Autodesk Fusion 360 part; units mm, degrees
(part 10 of 15)
  spline S14 degree 5 poles (-65.1777, -21.4619) (-65.1592, -21.4625) (-65.1224, -21.4637) (-65.0671, -21.4656) (-64.9935, -21.4682) (-64.9016, -21.4719) (-64.8097, -21.4758) (-64.7179, -21.48) (-64.6262, -21.4845) (-64.5346, -21.4894) (-64.443, -21.4945) (-64.3515, -21.4999) (-64.2602, -21.5056) (-64.1689, -21.5116) (-64.0777, -21.518) (-63.9866, -21.5246) (-63.8955, -21.5315) (-63.8046, -21.5388) (-63.7138, -21.5464) (-63.623, -21.5543) (-63.5324, -21.5625) (-63.4418, -21.571) (-63.3514, -21.5799) (-63.261, -21.5891) (-63.1708, -21.5986) (-63.0806, -21.6084) (-62.9906, -21.6186) (-62.9007, -21.6291) (-62.8108, -21.64) (-62.7211, -21.6512) (-62.6315, -21.6627) (-62.542, -21.6746) (-62.4527, -21.6869) (-62.3634, -21.6995) (-62.2743, -21.7125) (-62.1853, -21.7258) (-62.0964, -21.7395) (-62.0076, -21.7536) (-61.919, -21.768) (-61.8305, -21.7829) (-61.7422, -21.7981) (-61.654, -21.8137) (-61.5731, -21.8284) (-61.5099, -21.8401) (-61.4644, -21.8487) (-61.4364, -21.8541) (-61.4261, -21.8561) knots -1 -1 -1 -1 -1 -1 -0.985714 -0.971429 -0.957143 -0.942857 -0.928571 -0.914286 -0.9 -0.885714 -0.871429 -0.857143 -0.842857 -0.828571 -0.814286 -0.8 -0.785714 -0.771429 -0.757143 -0.742857 -0.728571 -0.714286 -0.7 -0.685714 -0.671429 -0.657143 -0.642857 -0.628571 -0.614286 -0.6 -0.585714 -0.571429 -0.557143 -0.542857 -0.528571 -0.514286 -0.5 -0.485714 -0.471429 -0.457143 -0.442857 -0.428571 -0.414286 -0.405839 -0.405839 -0.405839 -0.405839 -0.405839 -0.405839
  arc A14 (-60.836, -20.6774) -> (-61.4261, -21.8561) centre (2.0032, -52.8695) ccw
  spline S15 degree 5 poles (-60.836, -20.6774) (-60.8439, -20.6703) (-60.8649, -20.6511) (-60.8991, -20.6198) (-60.9463, -20.5763) (-61.0066, -20.5203) (-61.0719, -20.4591) (-61.137, -20.3975) (-61.202, -20.3355) (-61.2666, -20.2732) (-61.3311, -20.2106) (-61.3953, -20.1477) (-61.4593, -20.0844) (-61.5231, -20.0208) (-61.5867, -19.9569) (-61.6501, -19.8927) (-61.7132, -19.8282) (-61.7762, -19.7634) (-61.8389, -19.6983) (-61.9014, -19.6329) (-61.9637, -19.5672) (-62.0258, -19.5012) (-62.0877, -19.435) (-62.1494, -19.3684) (-62.2109, -19.3016) (-62.2722, -19.2345) (-62.3333, -19.1671) (-62.3942, -19.0995) (-62.4549, -19.0316) (-62.5154, -18.9634) (-62.5757, -18.8949) (-62.6359, -18.8262) (-62.6958, -18.7573) (-62.7555, -18.6881) (-62.815, -18.6186) (-62.8744, -18.5489) (-62.9335, -18.4789) (-62.9925, -18.4087) (-63.0512, -18.3382) (-63.1098, -18.2675) (-63.1682, -18.1965) (-63.2264, -18.1253) (-63.2844, -18.0539) (-63.3307, -17.9966) (-63.3653, -17.9535) (-63.3883, -17.9247) (-63.3998, -17.9103) knots 0.405839 0.405839 0.405839 0.405839 0.405839 0.405839 0.414286 0.428571 0.442857 0.457143 0.471429 0.485714 0.5 0.514286 0.528571 0.542857 0.557143 0.571429 0.585714 0.6 0.614286 0.628571 0.642857 0.657143 0.671429 0.685714 0.7 0.714286 0.728571 0.742857 0.757143 0.771429 0.785714 0.8 0.814286 0.828571 0.842857 0.857143 0.871429 0.885714 0.9 0.914286 0.928571 0.942857 0.957143 0.971429 0.985714 1 1 1 1 1 1
  arc A15 (-62.7659, -16.7493) -> (-63.3998, -17.9103) centre (2.0032, -52.8695) ccw
  spline S16 degree 5 poles (-62.7659, -16.7493) (-62.7476, -16.7512) (-62.7109, -16.755) (-62.6559, -16.7608) (-62.5827, -16.7687) (-62.4912, -16.7789) (-62.3999, -16.7894) (-62.3086, -16.8002) (-62.2174, -16.8112) (-62.1264, -16.8226) (-62.0354, -16.8342) (-61.9446, -16.8461) (-61.8539, -16.8583) (-61.7632, -16.8709) (-61.6727, -16.8837) (-61.5823, -16.8968) (-61.492, -16.9102) (-61.4018, -16.924) (-61.3118, -16.938) (-61.2218, -16.9523) (-61.132, -16.967) (-61.0423, -16.982) (-60.9527, -16.9973) (-60.8632, -17.0129) (-60.7739, -17.0288) (-60.6847, -17.0451) (-60.5956, -17.0616) (-60.5066, -17.0785) (-60.4178, -17.0958) (-60.3291, -17.1134) (-60.2406, -17.1313) (-60.1522, -17.1495) (-60.0639, -17.1681) (-59.9758, -17.1871) (-59.8878, -17.2063) (-59.8, -17.226) (-59.7123, -17.246) (-59.6248, -17.2664) (-59.5374, -17.2871) (-59.4502, -17.3082) (-59.3631, -17.3297) (-59.2763, -17.3516) (-59.1966, -17.372) (-59.1345, -17.3882) (-59.0897, -17.4) (-59.0622, -17.4074) (-59.052, -17.4101) knots -1 -1 -1 -1 -1 -1 -0.985714 -0.971429 -0.957143 -0.942857 -0.928571 -0.914286 -0.9 -0.885714 -0.871429 -0.857143 -0.842857 -0.828571 -0.814286 -0.8 -0.785714 -0.771429 -0.757143 -0.742857 -0.728571 -0.714286 -0.7 -0.685714 -0.671429 -0.657143 -0.642857 -0.628571 -0.614286 -0.6 -0.585714 -0.571429 -0.557143 -0.542857 -0.528571 -0.514286 -0.5 -0.485714 -0.471429 -0.457143 -0.442857 -0.428571 -0.414286 -0.405839 -0.405839 -0.405839 -0.405839 -0.405839 -0.405839
  arc A16 (-58.3794, -16.2765) -> (-59.052, -17.4101) centre (2.0032, -52.8695) ccw
  spline S17 degree 5 poles (-58.3794, -16.2765) (-58.3867, -16.2688) (-58.4063, -16.2482) (-58.4381, -16.2146) (-58.4822, -16.1678) (-58.5383, -16.1077) (-58.5991, -16.0419) (-58.6596, -15.9758) (-58.72, -15.9094) (-58.78, -15.8427) (-58.8399, -15.7756) (-58.8994, -15.7082) (-58.9588, -15.6406) (-59.0179, -15.5726) (-59.0767, -15.5043) (-59.1354, -15.4358) (-59.1937, -15.3669) (-59.2519, -15.2978) (-59.3098, -15.2284) (-59.3675, -15.1587) (-59.425, -15.0887) (-59.4822, -15.0185) (-59.5393, -14.9479) (-59.5961, -14.8772) (-59.6526, -14.8061) (-59.709, -14.7348) (-59.7651, -14.6633) (-59.821, -14.5914) (-59.8767, -14.5194) (-59.9322, -14.4471) (-59.9875, -14.3745) (-60.0426, -14.3017) (-60.0974, -14.2286) (-60.152, -14.1553) (-60.2065, -14.0818) (-60.2607, -14.008) (-60.3147, -13.934) (-60.3685, -13.8597) (-60.4221, -13.7852) (-60.4754, -13.7105) (-60.5286, -13.6356) (-60.5816, -13.5604) (-60.6344, -13.485) (-60.6764, -13.4246) (-60.7079, -13.3791) (-60.7288, -13.3487) (-60.7392, -13.3335) knots 0.405839 0.405839 0.405839 0.405839 0.405839 0.405839 0.414286 0.428571 0.442857 0.457143 0.471429 0.485714 0.5 0.514286 0.528571 0.542857 0.557143 0.571429 0.585714 0.6 0.614286 0.628571 0.642857 0.657143 0.671429 0.685714 0.7 0.714286 0.728571 0.742857 0.757143 0.771429 0.785714 0.8 0.814286 0.828571 0.842857 0.857143 0.871429 0.885714 0.9 0.914286 0.928571 0.942857 0.957143 0.971429 0.985714 1 1 1 1 1 1
  arc A17 (-60.0241, -12.2208) -> (-60.7392, -13.3335) centre (2.0032, -52.8695) ccw
  spline S18 degree 5 poles (-60.0241, -12.2208) (-60.0059, -12.224) (-59.9696, -12.2304) (-59.9152, -12.2401) (-59.8427, -12.2532) (-59.7522, -12.2699) (-59.6618, -12.2869) (-59.5716, -12.3041) (-59.4815, -12.3216) (-59.3914, -12.3394) (-59.3016, -12.3575) (-59.2118, -12.3759) (-59.1222, -12.3946) (-59.0327, -12.4135) (-58.9433, -12.4328) (-58.854, -12.4523) (-58.7649, -12.4721) (-58.676, -12.4923) (-58.5871, -12.5127) (-58.4984, -12.5334) (-58.4099, -12.5545) (-58.3215, -12.5758) (-58.2332, -12.5974) (-58.1451, -12.6194) (-58.0571, -12.6417) (-57.9693, -12.6642) (-57.8816, -12.6871) (-57.7941, -12.7103) (-57.7067, -12.7339) (-57.6195, -12.7577) (-57.5325, -12.7819) (-57.4456, -12.8064) (-57.3589, -12.8313) (-57.2723, -12.8564) (-57.1859, -12.882) (-57.0997, -12.9078) (-57.0137, -12.934) (-56.9278, -12.9606) (-56.8422, -12.9875) (-56.7567, -13.0148) (-56.6714, -13.0424) (-56.5863, -13.0704) (-56.5083, -13.0965) (-56.4475, -13.1171) (-56.4037, -13.1321) (-56.3768, -13.1414) (-56.3668, -13.1448) knots -1 -1 -1 -1 -1 -1 -0.985714 -0.971429 -0.957143 -0.942857 -0.928571 -0.914286 -0.9 -0.885714 -0.871429 -0.857143 -0.842857 -0.828571 -0.814286 -0.8 -0.785714 -0.771429 -0.757143 -0.742857 -0.728571 -0.714286 -0.7 -0.685714 -0.671429 -0.657143 -0.642857 -0.628571 -0.614286 -0.6 -0.585714 -0.571429 -0.557143 -0.542857 -0.528571 -0.514286 -0.5 -0.485714 -0.471429 -0.457143 -0.442857 -0.428571 -0.414286 -0.405839 -0.405839 -0.405839 -0.405839 -0.405839 -0.405839
  arc A18 (-55.615, -12.0621) -> (-56.3668, -13.1448) centre (2.0032, -52.8695) ccw
  spline S19 degree 5 poles (-55.615, -12.0621) (-55.6217, -12.0539) (-55.6398, -12.032) (-55.6692, -11.9961) (-55.7098, -11.9463) (-55.7614, -11.8824) (-55.8174, -11.8124) (-55.8731, -11.7422) (-55.9285, -11.6716) (-55.9837, -11.6008) (-56.0386, -11.5296) (-56.0932, -11.4582) (-56.1476, -11.3864) (-56.2017, -11.3144) (-56.2555, -11.2421) (-56.3091, -11.1696) (-56.3624, -11.0967) (-56.4155, -11.0236) (-56.4683, -10.9502) (-56.5209, -10.8766) (-56.5732, -10.8027) (-56.6253, -10.7286) (-56.6772, -10.6542) (-56.7288, -10.5795) (-56.7801, -10.5046) (-56.8313, -10.4295) (-56.8821, -10.3541) (-56.9328, -10.2785) (-56.9832, -10.2026) (-57.0334, -10.1265) (-57.0833, -10.0502) (-57.1331, -9.9736) (-57.1826, -9.8969) (-57.2318, -9.8198) (-57.2809, -9.7426) (-57.3297, -9.6651) (-57.3783, -9.5875) (-57.4266, -9.5096) (-57.4748, -9.4315) (-57.5227, -9.3531) (-57.5704, -9.2746) (-57.6179, -9.1958) (-57.6651, -9.1169) (-57.7027, -9.0535) (-57.7309, -9.006) (-57.7496, -8.9742) (-57.7589, -8.9583) knots 0.405839 0.405839 0.405839 0.405839 0.405839 0.405839 0.414286 0.428571 0.442857 0.457143 0.471429 0.485714 0.5 0.514286 0.528571 0.542857 0.557143 0.571429 0.585714 0.6 0.614286 0.628571 0.642857 0.657143 0.671429 0.685714 0.7 0.714286 0.728571 0.742857 0.757143 0.771429 0.785714 0.8 0.814286 0.828571 0.842857 0.857143 0.871429 0.885714 0.9 0.914286 0.928571 0.942857 0.957143 0.971429 0.985714 1 1 1 1 1 1
  arc A19 (-56.9662, -7.8993) -> (-57.7589, -8.9583) centre (2.0032, -52.8695) ccw
  spline S20 degree 5 poles (-56.9662, -7.8993) (-56.9483, -7.9038) (-56.9126, -7.9128) (-56.859, -7.9264) (-56.7876, -7.9447) (-56.6985, -7.9678) (-56.6096, -7.9911) (-56.5208, -8.0148) (-56.4321, -8.0387) (-56.3436, -8.0629) (-56.2553, -8.0873) (-56.167, -8.1121) (-56.079, -8.1371) (-55.991, -8.1624) (-55.9033, -8.1879) (-55.8157, -8.2138) (-55.7282, -8.2399) (-55.6409, -8.2664) (-55.5537, -8.2931) (-55.4667, -8.3201) (-55.3799, -8.3474) (-55.2932, -8.3749) (-55.2067, -8.4028) (-55.1204, -8.431) (-55.0342, -8.4595) (-54.9483, -8.4883) (-54.8624, -8.5174) (-54.7768, -8.5468) (-54.6913, -8.5765) (-54.606, -8.6065) (-54.5209, -8.6368) (-54.436, -8.6675) (-54.3513, -8.6984) (-54.2668, -8.7297) (-54.1824, -8.7613) (-54.0983, -8.7933) (-54.0144, -8.8256) (-53.9306, -8.8582) (-53.8471, -8.8911) (-53.7638, -8.9244) (-53.6807, -8.9581) (-53.5978, -8.9921) (-53.5219, -9.0236) (-53.4627, -9.0486) (-53.42, -9.0667) (-53.3938, -9.0778) (-53.3841, -9.082) knots -1 -1 -1 -1 -1 -1 -0.985714 -0.971429 -0.957143 -0.942857 -0.928571 -0.914286 -0.9 -0.885714 -0.871429 -0.857143 -0.842857 -0.828571 -0.814286 -0.8 -0.785714 -0.771429 -0.757143 -0.742857 -0.728571 -0.714286 -0.7 -0.685714 -0.671429 -0.657143 -0.642857 -0.628571 -0.614286 -0.6 -0.585714 -0.571429 -0.557143 -0.542857 -0.528571 -0.514286 -0.5 -0.485714 -0.471429 -0.457143 -0.442857 -0.428571 -0.414286 -0.405839 -0.405839 -0.405839 -0.405839 -0.405839 -0.405839
  arc A20 (-52.557, -8.0556) -> (-53.3841, -9.082) centre (2.0032, -52.8695) ccw
  spline S21 degree 5 poles (-52.557, -8.0556) (-52.5632, -8.047) (-52.5796, -8.0238) (-52.6064, -7.986) (-52.6433, -7.9334) (-52.6903, -7.8659) (-52.7411, -7.7922) (-52.7917, -7.7181) (-52.8419, -7.6438) (-52.8919, -7.5692) (-52.9416, -7.4943) (-52.9909, -7.4191) (-53.04, -7.3437) (-53.0889, -7.268) (-53.1374, -7.1921) (-53.1857, -7.1159) (-53.2337, -7.0394) (-53.2814, -6.9627) (-53.3289, -6.8857) (-53.3761, -6.8085) (-53.423, -6.7311) (-53.4696, -6.6534) (-53.516, -6.5755) (-53.5622, -6.4974) (-53.6081, -6.419) (-53.6537, -6.3404) (-53.6991, -6.2616) (-53.7442, -6.1826) (-53.7891, -6.1033) (-53.8337, -6.0238) (-53.8781, -5.9441) (-53.9222, -5.8642) (-53.9661, -5.7841) (-54.0098, -5.7037) (-54.0532, -5.6232) (-54.0963, -5.5425) (-54.1393, -5.4615) (-54.1819, -5.3804) (-54.2244, -5.299) (-54.2666, -5.2175) (-54.3086, -5.1357) (-54.3503, -5.0538) (-54.3918, -4.9717) (-54.4248, -4.9058) (-54.4495, -4.8563) (-54.4659, -4.8233) (-54.4741, -4.8068) knots 0.405839 0.405839 0.405839 0.405839 0.405839 0.405839 0.414286 0.428571 0.442857 0.457143 0.471429 0.485714 0.5 0.514286 0.528571 0.542857 0.557143 0.571429 0.585714 0.6 0.614286 0.628571 0.642857 0.657143 0.671429 0.685714 0.7 0.714286 0.728571 0.742857 0.757143 0.771429 0.785714 0.8 0.814286 0.828571 0.842857 0.857143 0.871429 0.885714 0.9 0.914286 0.928571 0.942857 0.957143 0.971429 0.985714 1 1 1 1 1 1
  arc A21 (-53.6078, -3.8071) -> (-54.4741, -4.8068) centre (2.0032, -52.8695) ccw
  spline S22 degree 5 poles (-53.6078, -3.8071) (-53.5903, -3.8128) (-53.5553, -3.8244) (-53.5028, -3.8417) (-53.4329, -3.865) (-53.3457, -3.8944) (-53.2587, -3.9241) (-53.1718, -3.954) (-53.0851, -3.9842) (-52.9985, -4.0146) (-52.9121, -4.0453) (-52.8259, -4.0763) (-52.7398, -4.1075) (-52.6539, -4.139) (-52.5682, -4.1708) (-52.4826, -4.2028) (-52.3973, -4.2351) (-52.3121, -4.2677) (-52.227, -4.3006) (-52.1422, -4.3337) (-52.0575, -4.3671) (-51.9731, -4.4008) (-51.8888, -4.4348) (-51.8047, -4.4691) (-51.7207, -4.5036) (-51.637, -4.5385) (-51.5535, -4.5736) (-51.4702, -4.6091) (-51.3871, -4.6448) (-51.3041, -4.6808) (-51.2214, -4.7171) (-51.1389, -4.7538) (-51.0566, -4.7907) (-50.9745, -4.8279) (-50.8927, -4.8655) (-50.811, -4.9033) (-50.7296, -4.9415) (-50.6484, -4.98) (-50.5674, -5.0189) (-50.4867, -5.058) (-50.4062, -5.0975) (-50.326, -5.1374) (-50.2525, -5.1742) (-50.1952, -5.2033) (-50.1539, -5.2244) (-50.1286, -5.2374) (-50.1192, -5.2422) knots -1 -1 -1 -1 -1 -1 -0.985714 -0.971429 -0.957143 -0.942857 -0.928571 -0.914286 -0.9 -0.885714 -0.871429 -0.857143 -0.842857 -0.828571 -0.814286 -0.8 -0.785714 -0.771429 -0.757143 -0.742857 -0.728571 -0.714286 -0.7 -0.685714 -0.671429 -0.657143 -0.642857 -0.628571 -0.614286 -0.6 -0.585714 -0.571429 -0.557143 -0.542857 -0.528571 -0.514286 -0.5 -0.485714 -0.471429 -0.457143 -0.442857 -0.428571 -0.414286 -0.405839 -0.405839 -0.405839 -0.405839 -0.405839 -0.405839
  arc A22 (-49.221, -4.2775) -> (-50.1192, -5.2422) centre (2.0032, -52.8695) ccw
  spline S23 degree 5 poles (-49.221, -4.2775) (-49.2265, -4.2685) (-49.2413, -4.2442) (-49.2653, -4.2045) (-49.2984, -4.1495) (-49.3404, -4.0788) (-49.3859, -4.0016) (-49.431, -3.9241) (-49.4758, -3.8464) (-49.5203, -3.7684) (-49.5645, -3.6902) (-49.6084, -3.6117) (-49.652, -3.533) (-49.6953, -3.454) (-49.7383, -3.3748) (-49.781, -3.2953) (-49.8235, -3.2156) (-49.8656, -3.1357) (-49.9074, -3.0556) (-49.949, -2.9752) (-49.9903, -2.8946) (-50.0313, -2.8138) (-50.072, -2.7328) (-50.1125, -2.6515) (-50.1527, -2.5701) (-50.1926, -2.4885) (-50.2322, -2.4066) (-50.2716, -2.3245) (-50.3107, -2.2423) (-50.3495, -2.1598) (-50.3881, -2.0771) (-50.4264, -1.9943) (-50.4645, -1.9112) (-50.5023, -1.828) (-50.5398, -1.7446) (-50.5771, -1.661) (-50.6142, -1.5772) (-50.651, -1.4932) (-50.6875, -1.409) (-50.7238, -1.3246) (-50.7598, -1.2401) (-50.7956, -1.1554) (-50.8311, -1.0705) (-50.8594, -1.0025) (-50.8804, -0.9514) (-50.8944, -0.9173) (-50.9014, -0.9002) knots 0.405839 0.405839 0.405839 0.405839 0.405839 0.405839 0.414286 0.428571 0.442857 0.457143 0.471429 0.485714 0.5 0.514286 0.528571 0.542857 0.557143 0.571429 0.585714 0.6 0.614286 0.628571 0.642857 0.657143 0.671429 0.685714 0.7 0.714286 0.728571 0.742857 0.757143 0.771429 0.785714 0.8 0.814286 0.828571 0.842857 0.857143 0.871429 0.885714 0.9 0.914286 0.928571 0.942857 0.957143 0.971429 0.985714 1 1 1 1 1 1
  arc A23 (-49.9661, 0.0351) -> (-50.9014, -0.9002) centre (2.0032, -52.8695) ccw
  spline S24 degree 5 poles (-49.9661, 0.0351) (-49.949, 0.0282) (-49.9149, 0.0142) (-49.8638, -0.0069) (-49.7957, -0.0351) (-49.7109, -0.0707) (-49.6261, -0.1065) (-49.5416, -0.1425) (-49.4573, -0.1788) (-49.3731, -0.2153) (-49.2891, -0.2521) (-49.2053, -0.2891) (-49.1217, -0.3264) (-49.0383, -0.364) (-48.955, -0.4018) (-48.872, -0.4398) (-48.7891, -0.4782) (-48.7065, -0.5167) (-48.624, -0.5556) (-48.5417, -0.5947) (-48.4597, -0.6341) (-48.3778, -0.6737) (-48.2962, -0.7136) (-48.2147, -0.7538) (-48.1335, -0.7942) (-48.0525, -0.835) (-47.9717, -0.876) (-47.8911, -0.9173) (-47.8107, -0.9588) (-47.7306, -1.0007) (-47.6506, -1.0428) (-47.571, -1.0852) (-47.4915, -1.1279) (-47.4123, -1.1709) (-47.3333, -1.2142) (-47.2546, -1.2578) (-47.1761, -1.3017) (-47.0978, -1.3459) (-47.0199, -1.3904) (-46.9421, -1.4353) (-46.8647, -1.4804) (-46.7875, -1.5259) (-46.7168, -1.5679) (-46.6617, -1.601) (-46.6221, -1.625) (-46.5978, -1.6397) (-46.5887, -1.6452) knots -1 -1 -1 -1 -1 -1 -0.985714 -0.971429 -0.957143 -0.942857 -0.928571 -0.914286 -0.9 -0.885714 -0.871429 -0.857143 -0.842857 -0.828571 -0.814286 -0.8 -0.785714 -0.771429 -0.757143 -0.742857 -0.728571 -0.714286 -0.7 -0.685714 -0.671429 -0.657143 -0.642857 -0.628571 -0.614286 -0.6 -0.585714 -0.571429 -0.557143 -0.542857 -0.528571 -0.514286 -0.5 -0.485714 -0.471429 -0.457143 -0.442857 -0.428571 -0.414286 -0.405839 -0.405839 -0.405839 -0.405839 -0.405839 -0.405839
  arc A24 (-45.624, -0.747) -> (-46.5887, -1.6452) centre (2.0032, -52.8695) ccw
  spline S25 degree 5 poles (-45.624, -0.747) (-45.6289, -0.7376) (-45.6419, -0.7123) (-45.663, -0.6711) (-45.692, -0.6138) (-45.7289, -0.5403) (-45.7687, -0.4601) (-45.8082, -0.3796) (-45.8474, -0.2988) (-45.8862, -0.2179) (-45.9247, -0.1367) (-45.9629, -0.0553) (-46.0008, 0.0264) (-46.0383, 0.1083) (-46.0756, 0.1903) (-46.1125, 0.2726) (-46.1491, 0.3551) (-46.1855, 0.4379) (-46.2215, 0.5208) (-46.2572, 0.6039) (-46.2926, 0.6872) (-46.3278, 0.7708) (-46.3626, 0.8545) (-46.3972, 0.9384) (-46.4314, 1.0225) (-46.4654, 1.1068) (-46.4991, 1.1913) (-46.5326, 1.2759) (-46.5657, 1.3608) (-46.5986, 1.4458) (-46.6311, 1.531) (-46.6635, 1.6164) (-46.6955, 1.7019) (-46.7273, 1.7877) (-46.7588, 1.8735) (-46.79, 1.9596) (-46.821, 2.0458) (-46.8517, 2.1322) (-46.8821, 2.2188) (-46.9123, 2.3055) (-46.9422, 2.3924) (-46.9718, 2.4794) (-47.0012, 2.5666) (-47.0245, 2.6365) (-47.0419, 2.689) (-47.0534, 2.724) (-47.0592, 2.7416) knots 0.405839 0.405839 0.405839 0.405839 0.405839 0.405839 0.414286 0.428571 0.442857 0.457143 0.471429 0.485714 0.5 0.514286 0.528571 0.542857 0.557143 0.571429 0.585714 0.6 0.614286 0.628571 0.642857 0.657143 0.671429 0.685714 0.7 0.714286 0.728571 0.742857 0.757143 0.771429 0.785714 0.8 0.814286 0.828571 0.842857 0.857143 0.871429 0.885714 0.9 0.914286 0.928571 0.942857 0.957143 0.971429 0.985714 1 1 1 1 1 1
  arc A25 (-46.0595, 3.6078) -> (-47.0592, 2.7416) centre (2.0032, -52.8695) ccw
  spline S26 degree 5 poles (-46.0595, 3.6078) (-46.043, 3.5996) (-46.0099, 3.5832) (-45.9605, 3.5586) (-45.8946, 3.5255) (-45.8125, 3.484) (-45.7305, 3.4423) (-45.6488, 3.4003) (-45.5672, 3.3581) (-45.4859, 3.3157) (-45.4047, 3.273) (-45.3238, 3.2301) (-45.2431, 3.1869) (-45.1625, 3.1435) (-45.0822, 3.0999) (-45.0021, 3.056) (-44.9222, 3.0118) (-44.8425, 2.9675) (-44.763, 2.9228) (-44.6837, 2.878) (-44.6047, 2.8328) (-44.5258, 2.7874) (-44.4472, 2.7418) (-44.3689, 2.6959) (-44.2907, 2.6498) (-44.2128, 2.6034) (-44.1352, 2.5567) (-44.0577, 2.5098) (-43.9805, 2.4626) (-43.9036, 2.4151) (-43.8269, 2.3674) (-43.7504, 2.3194) (-43.6742, 2.2711) (-43.5983, 2.2226) (-43.5226, 2.1738) (-43.4471, 2.1247) (-43.372, 2.0753) (-43.2971, 2.0256) (-43.2225, 1.9757) (-43.1481, 1.9254) (-43.0741, 1.8749) (-43.0003, 1.824) (-42.9329, 1.7771) (-42.8803, 1.7401) (-42.8425, 1.7134) (-42.8193, 1.6969) (-42.8106, 1.6908) knots -1 -1 -1 -1 -1 -1 -0.985714 -0.971429 -0.957143 -0.942857 -0.928571 -0.914286 -0.9 -0.885714 -0.871429 -0.857143 -0.842857 -0.828571 -0.814286 -0.8 -0.785714 -0.771429 -0.757143 -0.742857 -0.728571 -0.714286 -0.7 -0.685714 -0.671429 -0.657143 -0.642857 -0.628571 -0.614286 -0.6 -0.585714 -0.571429 -0.557143 -0.542857 -0.528571 -0.514286 -0.5 -0.485714 -0.471429 -0.457143 -0.442857 -0.428571 -0.414286 -0.405839 -0.405839 -0.405839 -0.405839 -0.405839 -0.405839
  arc A26 (-41.7843, 2.5179) -> (-42.8106, 1.6908) centre (2.0032, -52.8695) ccw
  spline S27 degree 5 poles (-41.7843, 2.5179) (-41.7885, 2.5276) (-41.7996, 2.5537) (-41.8177, 2.5964) (-41.8426, 2.6556) (-41.8742, 2.7315) (-41.9082, 2.8144) (-41.9418, 2.8975) (-41.9751, 2.9808) (-42.0081, 3.0644) (-42.0407, 3.1481) (-42.073, 3.232) (-42.1049, 3.3162) (-42.1365, 3.4005) (-42.1678, 3.485) (-42.1988, 3.5698) (-42.2295, 3.6547) (-42.2598, 3.7398) (-42.2898, 3.8251) (-42.3195, 3.9105) (-42.3489, 3.9962) (-42.378, 4.082) (-42.4068, 4.168) (-42.4353, 4.2541) (-42.4634, 4.3405) (-42.4913, 4.427) (-42.5189, 4.5136) (-42.5462, 4.6005) (-42.5732, 4.6875) (-42.5999, 4.7746) (-42.6263, 4.8619) (-42.6525, 4.9494) (-42.6783, 5.037) (-42.7039, 5.1248) (-42.7292, 5.2127) (-42.7542, 5.3008) (-42.7789, 5.389) (-42.8034, 5.4774) (-42.8276, 5.5659) (-42.8515, 5.6545) (-42.8751, 5.7433) (-42.8985, 5.8323) (-42.9216, 5.9213) (-42.9399, 5.9927) (-42.9534, 6.0463) (-42.9624, 6.0821) (-42.9669, 6.0999) knots 0.405839 0.405839 0.405839 0.405839 0.405839 0.405839 0.414286 0.428571 0.442857 0.457143 0.471429 0.485714 0.5 0.514286 0.528571 0.542857 0.557143 0.571429 0.585714 0.6 0.614286 0.628571 0.642857 0.657143 0.671429 0.685714 0.7 0.714286 0.728571 0.742857 0.757143 0.771429 0.785714 0.8 0.814286 0.828571 0.842857 0.857143 0.871429 0.885714 0.9 0.914286 0.928571 0.942857 0.957143 0.971429 0.985714 1 1 1 1 1 1
  arc A27 (-41.908, 6.8927) -> (-42.9669, 6.0999) centre (2.0032, -52.8695) ccw
  spline S28 degree 5 poles (-41.908, 6.8927) (-41.8921, 6.8833) (-41.8603, 6.8646) (-41.8127, 6.8365) (-41.7494, 6.7988) (-41.6704, 6.7516) (-41.5917, 6.7041) (-41.5131, 6.6564) (-41.4348, 6.6085) (-41.3567, 6.5604) (-41.2788, 6.512) (-41.2011, 6.4634) (-41.1237, 6.4146) (-41.0464, 6.3656) (-40.9694, 6.3163) (-40.8926, 6.2668) (-40.8161, 6.2171) (-40.7397, 6.1671) (-40.6636, 6.1169) (-40.5878, 6.0665) (-40.5122, 6.0159) (-40.4368, 5.965) (-40.3616, 5.9139) (-40.2867, 5.8625) (-40.2121, 5.8109) (-40.1377, 5.7591) (-40.0635, 5.707) (-39.9896, 5.6546) (-39.916, 5.6021) (-39.8426, 5.5492) (-39.7695, 5.4962) (-39.6967, 5.4428) (-39.6241, 5.3892) (-39.5518, 5.3354) (-39.4798, 5.2813) (-39.4081, 5.2269) (-39.3367, 5.1723) (-39.2655, 5.1174) (-39.1946, 5.0623) (-39.1241, 5.0069) (-39.0538, 4.9512) (-38.9839, 4.8952) (-38.9199, 4.8435) (-38.8701, 4.8029) (-38.8343, 4.7736) (-38.8123, 4.7555) (-38.8042, 4.7487) knots -1 -1 -1 -1 -1 -1 -0.985714 -0.971429 -0.957143 -0.942857 -0.928571 -0.914286 -0.9 -0.885714 -0.871429 -0.857143 -0.842857 -0.828571 -0.814286 -0.8 -0.785714 -0.771429 -0.757143 -0.742857 -0.728571 -0.714286 -0.7 -0.685714 -0.671429 -0.657143 -0.642857 -0.628571 -0.614286 -0.6 -0.585714 -0.571429 -0.557143 -0.542857 -0.528571 -0.514286 -0.5 -0.485714 -0.471429 -0.457143 -0.442857 -0.428571 -0.414286 -0.405839 -0.405839 -0.405839 -0.405839 -0.405839 -0.405839
  arc A28 (-37.7214, 5.5005) -> (-38.8042, 4.7487) centre (2.0032, -52.8695) ccw
  spline S29 degree 5 poles (-37.7214, 5.5005) (-37.7249, 5.5105) (-37.7342, 5.5374) (-37.7492, 5.5812) (-37.7698, 5.6421) (-37.7958, 5.72) (-37.8238, 5.8051) (-37.8515, 5.8904) (-37.8788, 5.9759) (-37.9057, 6.0616) (-37.9322, 6.1474) (-37.9584, 6.2335) (-37.9843, 6.3197) (-38.0098, 6.406) (-38.035, 6.4926) (-38.0599, 6.5793) (-38.0844, 6.6662) (-38.1086, 6.7532) (-38.1324, 6.8404) (-38.1559, 6.9278) (-38.1791, 7.0153) (-38.202, 7.103) (-38.2246, 7.1908) (-38.2469, 7.2788) (-38.2688, 7.3669) (-38.2905, 7.4552) (-38.3118, 7.5436) (-38.3328, 7.6322) (-38.3536, 7.7209) (-38.374, 7.8097) (-38.3941, 7.8987) (-38.414, 7.9878) (-38.4335, 8.077) (-38.4527, 8.1664) (-38.4717, 8.2559) (-38.4904, 8.3455) (-38.5087, 8.4353) (-38.5268, 8.5252) (-38.5446, 8.6152) (-38.5622, 8.7053) (-38.5794, 8.7956) (-38.5964, 8.886) (-38.613, 8.9764) (-38.6262, 9.0489) (-38.6359, 9.1034) (-38.6423, 9.1397) (-38.6455, 9.1578) knots 0.405839 0.405839 0.405839 0.405839 0.405839 0.405839 0.414286 0.428571 0.442857 0.457143 0.471429 0.485714 0.5 0.514286 0.528571 0.542857 0.557143 0.571429 0.585714 0.6 0.614286 0.628571 0.642857 0.657143 0.671429 0.685714 0.7 0.714286 0.728571 0.742857 0.757143 0.771429 0.785714 0.8 0.814286 0.828571 0.842857 0.857143 0.871429 0.885714 0.9 0.914286 0.928571 0.942857 0.957143 0.971429 0.985714 1 1 1 1 1 1
  arc A29 (-37.5327, 9.873) -> (-38.6455, 9.1578) centre (2.0032, -52.8695) ccw
  spline S30 degree 5 poles (-37.5327, 9.873) (-37.5175, 9.8625) (-37.4872, 9.8416) (-37.4417, 9.8101) (-37.3812, 9.7681) (-37.3058, 9.7153) (-37.2307, 9.6624) (-37.1557, 9.6092) (-37.081, 9.5558) (-37.0065, 9.5022) (-36.9323, 9.4484) (-36.8583, 9.3944) (-36.7845, 9.3402) (-36.711, 9.2858) (-36.6377, 9.2311) (-36.5646, 9.1763) (-36.4918, 9.1212) (-36.4192, 9.066) (-36.3469, 9.0105) (-36.2748, 8.9548) (-36.203, 8.8989) (-36.1314, 8.8427) (-36.0601, 8.7864) (-35.9891, 8.7298) (-35.9183, 8.673) (-35.8478, 8.616) (-35.7776, 8.5587) (-35.7076, 8.5013) (-35.6379, 8.4436) (-35.5685, 8.3856) (-35.4994, 8.3275) (-35.4305, 8.2691) (-35.3619, 8.2105) (-35.2937, 8.1516) (-35.2257, 8.0925) (-35.158, 8.0332) (-35.0907, 7.9736) (-35.0236, 7.9138) (-34.9569, 7.8537) (-34.8904, 7.7934) (-34.8243, 7.7328) (-34.7586, 7.672) (-34.6985, 7.6159) (-34.6517, 7.5719) (-34.618, 7.54) (-34.5974, 7.5204) (-34.5898, 7.5131) knots -1 -1 -1 -1 -1 -1 -0.985714 -0.971429 -0.957143 -0.942857 -0.928571 -0.914286 -0.9 -0.885714 -0.871429 -0.857143 -0.842857 -0.828571 -0.814286 -0.8 -0.785714 -0.771429 -0.757143 -0.742857 -0.728571 -0.714286 -0.7 -0.685714 -0.671429 -0.657143 -0.642857 -0.628571 -0.614286 -0.6 -0.585714 -0.571429 -0.557143 -0.542857 -0.528571 -0.514286 -0.5 -0.485714 -0.471429 -0.457143 -0.442857 -0.428571 -0.414286 -0.405839 -0.405839 -0.405839 -0.405839 -0.405839 -0.405839
  arc A30 (-33.4562, 8.1857) -> (-34.5898, 7.5131) centre (2.0032, -52.8695) ccw
  spline S31 degree 5 poles (-33.4562, 8.1857) (-33.4589, 8.1959) (-33.4662, 8.2234) (-33.4781, 8.2682) (-33.4943, 8.3304) (-33.5147, 8.41) (-33.5366, 8.4969) (-33.5581, 8.5839) (-33.5792, 8.6711) (-33.5999, 8.7585) (-33.6203, 8.846) (-33.6403, 8.9337) (-33.6599, 9.0215) (-33.6792, 9.1095) (-33.6982, 9.1976) (-33.7168, 9.2859) (-33.735, 9.3743) (-33.7529, 9.4629) (-33.7705, 9.5515) (-33.7877, 9.6404) (-33.8046, 9.7293) (-33.8212, 9.8184) (-33.8375, 9.9076) (-33.8534, 9.997) (-33.869, 10.0864) (-33.8843, 10.176) (-33.8993, 10.2657) (-33.9139, 10.3556) (-33.9283, 10.4455) (-33.9423, 10.5356) (-33.956, 10.6258) (-33.9695, 10.716) (-33.9826, 10.8065) (-33.9954, 10.897) (-34.0079, 10.9876) (-34.0202, 11.0783) (-34.0321, 11.1692) (-34.0437, 11.2601) (-34.0551, 11.3512) (-34.0661, 11.4423) (-34.0769, 11.5336) (-34.0873, 11.6249) (-34.0975, 11.7164) (-34.1054, 11.7896) (-34.1113, 11.8446) (-34.1151, 11.8813) (-34.117, 11.8996) knots 0.405839 0.405839 0.405839 0.405839 0.405839 0.405839 0.414286 0.428571 0.442857 0.457143 0.471429 0.485714 0.5 0.514286 0.528571 0.542857 0.557143 0.571429 0.585714 0.6 0.614286 0.628571 0.642857 0.657143 0.671429 0.685714 0.7 0.714286 0.728571 0.742857 0.757143 0.771429 0.785714 0.8 0.814286 0.828571 0.842857 0.857143 0.871429 0.885714 0.9 0.914286 0.928571 0.942857 0.957143 0.971429 0.985714 1 1 1 1 1 1
  arc A31 (-32.956, 12.5336) -> (-34.117, 11.8996) centre (2.0032, -52.8695) ccw
  spline S32 degree 5 poles (-32.956, 12.5336) (-32.9416, 12.5221) (-32.9128, 12.499) (-32.8697, 12.4644) (-32.8124, 12.4182) (-32.7409, 12.3601) (-32.6697, 12.3019) (-32.5988, 12.2436) (-32.5281, 12.185) (-32.4576, 12.1262) (-32.3874, 12.0673) (-32.3174, 12.0081) (-32.2477, 11.9488) (-32.1782, 11.8892) (-32.109, 11.8295) (-32.04, 11.7696) (-31.9713, 11.7095) (-31.9029, 11.6492) (-31.8347, 11.5887) (-31.7668, 11.528) (-31.6992, 11.4671) (-31.6318, 11.406) (-31.5647, 11.3447) (-31.4979, 11.2832) (-31.4313, 11.2215) (-31.365, 11.1596) (-31.2991, 11.0975) (-31.2334, 11.0352) (-31.168, 10.9726) (-31.1029, 10.9099) (-31.0381, 10.847) (-30.9736, 10.7838) (-30.9093, 10.7204) (-30.8455, 10.6569) (-30.7819, 10.5931) (-30.7186, 10.5291) (-30.6557, 10.4648) (-30.593, 10.4004) (-30.5308, 10.3357) (-30.4688, 10.2708) (-30.4072, 10.2057) (-30.3459, 10.1403) (-30.29, 10.0801) (-30.2465, 10.0328) (-30.2152, 9.9986) (-30.196, 9.9776) (-30.1889, 9.9698) knots -1 -1 -1 -1 -1 -1 -0.985714 -0.971429 -0.957143 -0.942857 -0.928571 -0.914286 -0.9 -0.885714 -0.871429 -0.857143 -0.842857 -0.828571 -0.814286 -0.8 -0.785714 -0.771429 -0.757143 -0.742857 -0.728571 -0.714286 -0.7 -0.685714 -0.671429 -0.657143 -0.642857 -0.628571 -0.614286 -0.6 -0.585714 -0.571429 -0.557143 -0.542857 -0.528571 -0.514286 -0.5 -0.485714 -0.471429 -0.457143 -0.442857 -0.428571 -0.414286 -0.405839 -0.405839 -0.405839 -0.405839 -0.405839 -0.405839
  arc A32 (-29.0102, 10.5598) -> (-30.1889, 9.9698) centre (2.0032, -52.8695) ccw
  spline S33 degree 5 poles (-29.0102, 10.5598) (-29.0122, 10.5702) (-29.0175, 10.5981) (-29.0261, 10.6436) (-29.0379, 10.7068) (-29.0526, 10.7877) (-29.0682, 10.8759) (-29.0834, 10.9643) (-29.0982, 11.0528) (-29.1127, 11.1414) (-29.1268, 11.2301) (-29.1405, 11.319) (-29.1538, 11.408) (-29.1668, 11.4972) (-29.1794, 11.5864) (-29.1916, 11.6758) (-29.2035, 11.7653) (-29.2151, 11.8549) (-29.2263, 11.9446) (-29.2371, 12.0344) (-29.2477, 12.1243) (-29.2578, 12.2144) (-29.2677, 12.3045) (-29.2772, 12.3948) (-29.2864, 12.4851) (-29.2952, 12.5756) (-29.3038, 12.6661) (-29.312, 12.7568) (-29.3199, 12.8475) (-29.3275, 12.9383) (-29.3347, 13.0293) (-29.3417, 13.1203) (-29.3483, 13.2114) (-29.3546, 13.3026) (-29.3607, 13.3939) (-29.3664, 13.4853) (-29.3718, 13.5767) (-29.3769, 13.6683) (-29.3817, 13.7599) (-29.3862, 13.8516) (-29.3905, 13.9434) (-29.3944, 14.0353) (-29.398, 14.1272) (-29.4007, 14.2009) (-29.4026, 14.2561) (-29.4038, 14.293) (-29.4044, 14.3114) knots 0.405839 0.405839 0.405839 0.405839 0.405839 0.405839 0.414286 0.428571 0.442857 0.457143 0.471429 0.485714 0.5 0.514286 0.528571 0.542857 0.557143 0.571429 0.585714 0.6 0.614286 0.628571 0.642857 0.657143 0.671429 0.685714 0.7 0.714286 0.728571 0.742857 0.757143 0.771429 0.785714 0.8 0.814286 0.828571 0.842857 0.857143 0.871429 0.885714 0.9 0.914286 0.928571 0.942857 0.957143 0.971429 0.985714 1 1 1 1 1 1
  arc A33 (-28.2011, 14.8609) -> (-29.4044, 14.3114) centre (2.0032, -52.8695) ccw
  spline S34 degree 5 poles (-28.2011, 14.8609) (-28.1876, 14.8484) (-28.1605, 14.8234) (-28.12, 14.7858) (-28.0661, 14.7355) (-27.999, 14.6726) (-27.9321, 14.6094) (-27.8655, 14.5461) (-27.7992, 14.4827) (-27.7331, 14.419) (-27.6672, 14.3552) (-27.6017, 14.2912) (-27.5363, 14.227) (-27.4713, 14.1627) (-27.4065, 14.0982) (-27.342, 14.0335) (-27.2778, 13.9687) (-27.2138, 13.9036) (-27.1501, 13.8384) (-27.0867, 13.773) (-27.0236, 13.7075) (-26.9607, 13.6417) (-26.8982, 13.5758) (-26.8359, 13.5097) (-26.7739, 13.4434) (-26.7122, 13.3769) (-26.6509, 13.3102) (-26.5898, 13.2434) (-26.529, 13.1764) (-26.4685, 13.1092) (-26.4084, 13.0418) (-26.3486, 12.9742) (-26.289, 12.9064) (-26.2298, 12.8384) (-26.171, 12.7702) (-26.1124, 12.7019) (-26.0542, 12.6333) (-25.9964, 12.5646) (-25.9389, 12.4956) (-25.8817, 12.4264) (-25.8249, 12.3571) (-25.7684, 12.2875) (-25.7169, 12.2234) (-25.6769, 12.1732) (-25.6481, 12.1369) (-25.6305, 12.1145) (-25.624, 12.1062) knots -1 -1 -1 -1 -1 -1 -0.985714 -0.971429 -0.957143 -0.942857 -0.928571 -0.914286 -0.9 -0.885714 -0.871429 -0.857143 -0.842857 -0.828571 -0.814286 -0.8 -0.785714 -0.771429 -0.757143 -0.742857 -0.728571 -0.714286 -0.7 -0.685714 -0.671429 -0.657143 -0.642857 -0.628571 -0.614286 -0.6 -0.585714 -0.571429 -0.557143 -0.542857 -0.528571 -0.514286 -0.5 -0.485714 -0.471429 -0.457143 -0.442857 -0.428571 -0.414286 -0.405839 -0.405839 -0.405839 -0.405839 -0.405839 -0.405839
  arc A34 (-24.4062, 12.6106) -> (-25.624, 12.1062) centre (2.0032, -52.8695) ccw
  spline S35 degree 5 poles (-24.4062, 12.6106) (-24.4074, 12.6211) (-24.4108, 12.6494) (-24.4161, 12.6954) (-24.4233, 12.7593) (-24.4322, 12.841) (-24.4415, 12.9301) (-24.4504, 13.0193) (-24.4588, 13.1086) (-24.4669, 13.1981) (-24.4746, 13.2876) (-24.482, 13.3772) (-24.4889, 13.467) (-24.4955, 13.5568) (-24.5017, 13.6467) (-24.5075, 13.7367) (-24.513, 13.8268) (-24.5182, 13.917) (-24.5229, 14.0073) (-24.5273, 14.0977) (-24.5314, 14.1881) (-24.5352, 14.2787) (-24.5385, 14.3693) (-24.5416, 14.46) (-24.5443, 14.5508) (-24.5467, 14.6416) (-24.5488, 14.7326) (-24.5505, 14.8236) (-24.5519, 14.9146) (-24.553, 15.0058) (-24.5537, 15.097) (-24.5542, 15.1883) (-24.5543, 15.2796) (-24.5541, 15.3711) (-24.5536, 15.4625) (-24.5528, 15.5541) (-24.5516, 15.6457) (-24.5502, 15.7374) (-24.5485, 15.8291) (-24.5464, 15.9209) (-24.5441, 16.0128) (-24.5415, 16.1047) (-24.5385, 16.1967) (-24.536, 16.2703) (-24.5339, 16.3256) (-24.5324, 16.3624) (-24.5317, 16.3808) knots 0.405839 0.405839 0.405839 0.405839 0.405839 0.405839 0.414286 0.428571 0.442857 0.457143 0.471429 0.485714 0.5 0.514286 0.528571 0.542857 0.557143 0.571429 0.585714 0.6 0.614286 0.628571 0.642857 0.657143 0.671429 0.685714 0.7 0.714286 0.728571 0.742857 0.757143 0.771429 0.785714 0.8 0.814286 0.828571 0.842857 0.857143 0.871429 0.885714 0.9 0.914286 0.928571 0.942857 0.957143 0.971429 0.985714 1 1 1 1 1 1
  arc A35 (-23.2923, 16.8431) -> (-24.5317, 16.3808) centre (2.0032, -52.8695) ccw
  spline S36 degree 5 poles (-23.2923, 16.8431) (-23.2797, 16.8296) (-23.2545, 16.8027) (-23.2168, 16.7623) (-23.1666, 16.7084) (-23.1041, 16.6408) (-23.042, 16.5731) (-22.98, 16.5052) (-22.9184, 16.4371) (-22.857, 16.3689) (-22.7959, 16.3006) (-22.735, 16.2321) (-22.6745, 16.1634) (-22.6142, 16.0946) (-22.5542, 16.0256) (-22.4944, 15.9565) (-22.435, 15.8872) (-22.3758, 15.8178) (-22.3169, 15.7482) (-22.2584, 15.6785) (-22.2001, 15.6086) (-22.1421, 15.5385) (-22.0844, 15.4683) (-22.027, 15.3979) (-21.9699, 15.3274) (-21.9131, 15.2566) (-21.8566, 15.1858) (-21.8005, 15.1148) (-21.7447, 15.0436) (-21.6891, 14.9722) (-21.634, 14.9007) (-21.5791, 14.829) (-21.5246, 14.7571) (-21.4704, 14.6851) (-21.4165, 14.6129) (-21.363, 14.5405) (-21.3098, 14.468) (-21.257, 14.3953) (-21.2046, 14.3224) (-21.1525, 14.2494) (-21.1008, 14.1761) (-21.0494, 14.1027) (-21.0026, 14.0351) (-20.9663, 13.9821) (-20.9402, 13.9439) (-20.9242, 13.9203) (-20.9183, 13.9116) knots -1 -1 -1 -1 -1 -1 -0.985714 -0.971429 -0.957143 -0.942857 -0.928571 -0.914286 -0.9 -0.885714 -0.871429 -0.857143 -0.842857 -0.828571 -0.814286 -0.8 -0.785714 -0.771429 -0.757143 -0.742857 -0.728571 -0.714286 -0.7 -0.685714 -0.671429 -0.657143 -0.642857 -0.628571 -0.614286 -0.6 -0.585714 -0.571429 -0.557143 -0.542857 -0.528571 -0.514286 -0.5 -0.485714 -0.471429 -0.457143 -0.442857 -0.428571 -0.414286 -0.405839 -0.405839 -0.405839 -0.405839 -0.405839 -0.405839
  arc A36 (-19.6676, 14.3278) -> (-20.9183, 13.9116) centre (2.0032, -52.8695) ccw
  spline S37 degree 5 poles (-19.6676, 14.3278) (-19.6681, 14.3384) (-19.6694, 14.3668) (-19.6715, 14.4131) (-19.6741, 14.4773) (-19.6771, 14.5594) (-19.68, 14.649) (-19.6825, 14.7386) (-19.6846, 14.8283) (-19.6863, 14.9181) (-19.6876, 15.0079) (-19.6885, 15.0979) (-19.689, 15.1879) (-19.6892, 15.2779) (-19.689, 15.3681) (-19.6884, 15.4583) (-19.6874, 15.5486) (-19.6861, 15.6389) (-19.6844, 15.7293) (-19.6824, 15.8197) (-19.68, 15.9102) (-19.6772, 16.0008) (-19.6742, 16.0914) (-19.6707, 16.1821) (-19.667, 16.2729) (-19.6629, 16.3637) (-19.6584, 16.4545) (-19.6537, 16.5454) (-19.6486, 16.6363) (-19.6431, 16.7273) (-19.6374, 16.8184) (-19.6313, 16.9095) (-19.6249, 17.0006) (-19.6182, 17.0918) (-19.6112, 17.183) (-19.6038, 17.2742) (-19.5962, 17.3655) (-19.5882, 17.4569) (-19.5799, 17.5483) (-19.5713, 17.6397) (-19.5625, 17.7312) (-19.5533, 17.8226) (-19.5438, 17.9142) (-19.536, 17.9874) (-19.53, 18.0424) (-19.5259, 18.079) (-19.5238, 18.0974) knots 0.405839 0.405839 0.405839 0.405839 0.405839 0.405839 0.414286 0.428571 0.442857 0.457143 0.471429 0.485714 0.5 0.514286 0.528571 0.542857 0.557143 0.571429 0.585714 0.6 0.614286 0.628571 0.642857 0.657143 0.671429 0.685714 0.7 0.714286 0.728571 0.742857 0.757143 0.771429 0.785714 0.8 0.814286 0.828571 0.842857 0.857143 0.871429 0.885714 0.9 0.914286 0.928571 0.942857 0.957143 0.971429 0.985714 1 1 1 1 1 1
  arc A37 (-18.2546, 18.47) -> (-19.5238, 18.0974) centre (2.0032, -52.8695) ccw
  spline S38 degree 5 poles (-18.2546, 18.47) (-18.243, 18.4557) (-18.2198, 18.4271) (-18.185, 18.3841) (-18.1388, 18.3267) (-18.0814, 18.2548) (-18.0242, 18.1828) (-17.9672, 18.1107) (-17.9106, 18.0384) (-17.8542, 17.966) (-17.7982, 17.8935) (-17.7424, 17.8208) (-17.6868, 17.748) (-17.6316, 17.6751) (-17.5767, 17.602) (-17.522, 17.5288) (-17.4677, 17.4555) (-17.4136, 17.382) (-17.3598, 17.3084) (-17.3064, 17.2346) (-17.2532, 17.1607) (-17.2004, 17.0867) (-17.1478, 17.0126) (-17.0956, 16.9383) (-17.0437, 16.8638) (-16.9921, 16.7892) (-16.9409, 16.7145) (-16.8899, 16.6397) (-16.8393, 16.5647) (-16.789, 16.4895) (-16.7391, 16.4143) (-16.6895, 16.3388) (-16.6402, 16.2633) (-16.5913, 16.1876) (-16.5427, 16.1117) (-16.4945, 16.0357) (-16.4466, 15.9596) (-16.3991, 15.8833) (-16.352, 15.8068) (-16.3053, 15.7303) (-16.2589, 15.6535) (-16.213, 15.5766) (-16.1711, 15.5059) (-16.1386, 15.4504) (-16.1153, 15.4104) (-16.101, 15.3858) (-16.0958, 15.3766) knots -1 -1 -1 -1 -1 -1 -0.985714 -0.971429 -0.957143 -0.942857 -0.928571 -0.914286 -0.9 -0.885714 -0.871429 -0.857143 -0.842857 -0.828571 -0.814286 -0.8 -0.785714 -0.771429 -0.757143 -0.742857 -0.728571 -0.714286 -0.7 -0.685714 -0.671429 -0.657143 -0.642857 -0.628571 -0.614286 -0.6 -0.585714 -0.571429 -0.557143 -0.542857 -0.528571 -0.514286 -0.5 -0.485714 -0.471429 -0.457143 -0.442857 -0.428571 -0.414286 -0.405839 -0.405839 -0.405839 -0.405839 -0.405839 -0.405839
  arc A38 (-14.8186, 15.7026) -> (-16.0958, 15.3766) centre (2.0032, -52.8695) ccw
  spline S39 degree 5 poles (-14.8186, 15.7026) (-14.8183, 15.7132) (-14.8176, 15.7416) (-14.8163, 15.7879) (-14.8144, 15.8522) (-14.8116, 15.9343) (-14.8081, 16.0238) (-14.8041, 16.1134) (-14.7998, 16.203) (-14.7951, 16.2927) (-14.79, 16.3824) (-14.7845, 16.4722) (-14.7786, 16.562) (-14.7723, 16.6518) (-14.7657, 16.7417) (-14.7586, 16.8317) (-14.7513, 16.9216) (-14.7435, 17.0116) (-14.7354, 17.1017) (-14.7269, 17.1918) (-14.718, 17.2819) (-14.7089, 17.372) (-14.6993, 17.4622) (-14.6894, 17.5524) (-14.6792, 17.6426) (-14.6686, 17.7329) (-14.6577, 17.8232) (-14.6465, 17.9135) (-14.6349, 18.0039) (-14.623, 18.0942) (-14.6108, 18.1846) (-14.5982, 18.2751) (-14.5853, 18.3655) (-14.5721, 18.456) (-14.5586, 18.5465) (-14.5448, 18.637) (-14.5306, 18.7275) (-14.5162, 18.818) (-14.5014, 18.9086) (-14.4863, 18.9992) (-14.4709, 19.0897) (-14.4552, 19.1804) (-14.4392, 19.271) (-14.4262, 19.3435) (-14.4163, 19.3979) (-14.4096, 19.4341) (-14.4063, 19.4523) knots 0.405839 0.405839 0.405839 0.405839 0.405839 0.405839 0.414286 0.428571 0.442857 0.457143 0.471429 0.485714 0.5 0.514286 0.528571 0.542857 0.557143 0.571429 0.585714 0.6 0.614286 0.628571 0.642857 0.657143 0.671429 0.685714 0.7 0.714286 0.728571 0.742857 0.757143 0.771429 0.785714 0.8 0.814286 0.828571 0.842857 0.857143 0.871429 0.885714 0.9 0.914286 0.928571 0.942857 0.957143 0.971429 0.985714 1 1 1 1 1 1
  arc A39 (-13.1137, 19.7334) -> (-14.4063, 19.4523) centre (2.0032, -52.8695) ccw
  spline S40 degree 5 poles (-13.1137, 19.7334) (-13.1031, 19.7183) (-13.082, 19.6881) (-13.0504, 19.6428) (-13.0084, 19.5822) (-12.9562, 19.5064) (-12.9043, 19.4305) (-12.8527, 19.3545) (-12.8014, 19.2784) (-12.7503, 19.2022) (-12.6995, 19.1258) (-12.6491, 19.0493) (-12.5989, 18.9728) (-12.549, 18.8961) (-12.4994, 18.8193) (-12.4501, 18.7423) (-12.4011, 18.6653) (-12.3524, 18.5882) (-12.3041, 18.5109) (-12.256, 18.4335) (-12.2083, 18.356) (-12.1608, 18.2784) (-12.1137, 18.2007) (-12.0669, 18.1229) (-12.0205, 18.0449) (-11.9743, 17.9669) (-11.9285, 17.8887) (-11.883, 17.8104) (-11.8379, 17.732) (-11.7931, 17.6534) (-11.7487, 17.5748) (-11.7046, 17.496) (-11.6608, 17.4171) (-11.6174, 17.3381) (-11.5744, 17.259) (-11.5317, 17.1798) (-11.4894, 17.1004) (-11.4475, 17.0209) (-11.406, 16.9413) (-11.3648, 16.8616) (-11.324, 16.7817) (-11.2837, 16.7018) (-11.2469, 16.6282) (-11.2185, 16.5706) (-11.1981, 16.529) (-11.1856, 16.5034) (-11.181, 16.4939) knots -1 -1 -1 -1 -1 -1 -0.985714 -0.971429 -0.957143 -0.942857 -0.928571 -0.914286 -0.9 -0.885714 -0.871429 -0.857143 -0.842857 -0.828571 -0.814286 -0.8 -0.785714 -0.771429 -0.757143 -0.742857 -0.728571 -0.714286 -0.7 -0.685714 -0.671429 -0.657143 -0.642857 -0.628571 -0.614286 -0.6 -0.585714 -0.571429 -0.557143 -0.542857 -0.528571 -0.514286 -0.5 -0.485714 -0.471429 -0.457143 -0.442857 -0.428571 -0.414286 -0.405839 -0.405839 -0.405839 -0.405839 -0.405839 -0.405839
  arc A40 (-9.8838, 16.7279) -> (-11.181, 16.4939) centre (2.0032, -52.8695) ccw
  spline S41 degree 5 poles (-9.8838, 16.7279) (-9.8828, 16.7385) (-9.8801, 16.7668) (-9.8755, 16.8129) (-9.869, 16.8768) (-9.8603, 16.9586) (-9.8504, 17.0476) (-9.8401, 17.1367) (-9.8294, 17.2257) (-9.8183, 17.3149) (-9.8068, 17.404) (-9.7949, 17.4931) (-9.7827, 17.5823) (-9.77, 17.6714) (-9.7569, 17.7606) (-9.7435, 17.8498) (-9.7297, 17.9391) (-9.7156, 18.0283) (-9.701, 18.1175) (-9.6861, 18.2068) (-9.6709, 18.296) (-9.6553, 18.3853) (-9.6394, 18.4745) (-9.6231, 18.5638) (-9.6064, 18.6531) (-9.5894, 18.7424) (-9.5721, 18.8317) (-9.5545, 18.921) (-9.5365, 19.0102) (-9.5181, 19.0995) (-9.4995, 19.1888) (-9.4805, 19.2781) (-9.4612, 19.3674) (-9.4416, 19.4567) (-9.4217, 19.546) (-9.4014, 19.6353) (-9.3808, 19.7246) (-9.3599, 19.8138) (-9.3387, 19.9031) (-9.3172, 19.9924) (-9.2954, 20.0817) (-9.2733, 20.1709) (-9.2509, 20.2602) (-9.2327, 20.3316) (-9.219, 20.3851) (-9.2097, 20.4208) (-9.2051, 20.4386) knots 0.405839 0.405839 0.405839 0.405839 0.405839 0.405839 0.414286 0.428571 0.442857 0.457143 0.471429 0.485714 0.5 0.514286 0.528571 0.542857 0.557143 0.571429 0.585714 0.6 0.614286 0.628571 0.642857 0.657143 0.671429 0.685714 0.7 0.714286 0.728571 0.742857 0.757143 0.771429 0.785714 0.8 0.814286 0.828571 0.842857 0.857143 0.871429 0.885714 0.9 0.914286 0.928571 0.942857 0.957143 0.971429 0.985714 1 1 1 1 1 1
  arc A41 (-7.8958, 20.6269) -> (-9.2051, 20.4386) centre (2.0032, -52.8695) ccw
  spline S42 degree 5 poles (-7.8958, 20.6269) (-7.8863, 20.6111) (-7.8674, 20.5794) (-7.8391, 20.5319) (-7.8015, 20.4685) (-7.7549, 20.3892) (-7.7085, 20.3098) (-7.6624, 20.2303) (-7.6167, 20.1507) (-7.5712, 20.071) (-7.526, 19.9913) (-7.4811, 19.9114) (-7.4365, 19.8314) (-7.3922, 19.7514) (-7.3482, 19.6712) (-7.3046, 19.591) (-7.2612, 19.5106) (-7.2181, 19.4302) (-7.1754, 19.3497) (-7.133, 19.2691) (-7.0909, 19.1884) (-7.0491, 19.1076) (-7.0077, 19.0267) (-6.9665, 18.9458) (-6.9258, 18.8647) (-6.8853, 18.7835) (-6.8452, 18.7023) (-6.8054, 18.6209) (-6.766, 18.5395) (-6.7269, 18.458) (-6.6882, 18.3764) (-6.6498, 18.2946) (-6.6118, 18.2128) (-6.5742, 18.1309) (-6.5369, 18.0489) (-6.5, 17.9669) (-6.4634, 17.8847) (-6.4273, 17.8024) (-6.3915, 17.72) (-6.3562, 17.6376) (-6.3212, 17.555) (-6.2866, 17.4724) (-6.2553, 17.3964) (-6.231, 17.3369) (-6.2136, 17.2939) (-6.203, 17.2675) (-6.1991, 17.2577) knots -1 -1 -1 -1 -1 -1 -0.985714 -0.971429 -0.957143 -0.942857 -0.928571 -0.914286 -0.9 -0.885714 -0.871429 -0.857143 -0.842857 -0.828571 -0.814286 -0.8 -0.785714 -0.771429 -0.757143 -0.742857 -0.728571 -0.714286 -0.7 -0.685714 -0.671429 -0.657143 -0.642857 -0.628571 -0.614286 -0.6 -0.585714 -0.571429 -0.557143 -0.542857 -0.528571 -0.514286 -0.5 -0.485714 -0.471429 -0.457143 -0.442857 -0.428571 -0.414286 -0.405839 -0.405839 -0.405839 -0.405839 -0.405839 -0.405839
  arc A42 (-4.8885, 17.3986) -> (-6.1991, 17.2577) centre (2.0032, -52.8695) ccw
  spline S43 degree 5 poles (-4.8885, 17.3986) (-4.8868, 17.409) (-4.882, 17.4371) (-4.8742, 17.4828) (-4.8631, 17.5461) (-4.8486, 17.627) (-4.8324, 17.7151) (-4.8158, 17.8032) (-4.7988, 17.8913) (-4.7813, 17.9794) (-4.7635, 18.0674) (-4.7453, 18.1555) (-4.7267, 18.2436) (-4.7077, 18.3316) (-4.6883, 18.4196) (-4.6685, 18.5077) (-4.6484, 18.5957) (-4.6279, 18.6836) (-4.6071, 18.7716) (-4.5858, 18.8596) (-4.5643, 18.9475) (-4.5423, 19.0354) (-4.5201, 19.1233) (-4.4974, 19.2112) (-4.4745, 19.2991) (-4.4512, 19.3869) (-4.4275, 19.4747) (-4.4035, 19.5626) (-4.3792, 19.6503) (-4.3546, 19.7381) (-4.3296, 19.8258) (-4.3043, 19.9135) (-4.2787, 20.0012) (-4.2527, 20.0889) (-4.2265, 20.1765) (-4.1999, 20.2641) (-4.173, 20.3517) (-4.1458, 20.4393) (-4.1183, 20.5268) (-4.0905, 20.6143) (-4.0624, 20.7018) (-4.034, 20.7893) (-4.0052, 20.8767) (-3.982, 20.9466) (-3.9645, 20.999) (-3.9527, 21.034) (-3.9468, 21.0514) knots 0.405839 0.405839 0.405839 0.405839 0.405839 0.405839 0.414286 0.428571 0.442857 0.457143 0.471429 0.485714 0.5 0.514286 0.528571 0.542857 0.557143 0.571429 0.585714 0.6 0.614286 0.628571 0.642857 0.657143 0.671429 0.685714 0.7 0.714286 0.728571 0.742857 0.757143 0.771429 0.785714 0.8 0.814286 0.828571 0.842857 0.857143 0.871429 0.885714 0.9 0.914286 0.928571 0.942857 0.957143 0.971429 0.985714 1 1 1 1 1 1
  arc A43 (-2.6274, 21.1458) -> (-3.9468, 21.0514) centre (2.0032, -52.8695) ccw
  spline S44 degree 5 poles (-2.6274, 21.1458) (-2.6191, 21.1294) (-2.6024, 21.0964) (-2.5776, 21.0471) (-2.5447, 20.9812) (-2.5038, 20.8987) (-2.4632, 20.8162) (-2.4229, 20.7336) (-2.383, 20.6509) (-2.3433, 20.5682) (-2.3039, 20.4854) (-2.2648, 20.4025) (-2.226, 20.3196) (-2.1876, 20.2366) (-2.1494, 20.1535) (-2.1116, 20.0704) (-2.074, 19.9871) (-2.0368, 19.9039) (-2, 19.8205) (-1.9634, 19.7371) (-1.9272, 19.6536) (-1.8913, 19.57) (-1.8557, 19.4864) (-1.8205, 19.4027) (-1.7855, 19.3189) (-1.751, 19.2351) (-1.7168, 19.1512) (-1.6829, 19.0672) (-1.6494, 18.9832) (-1.6162, 18.899) (-1.5834, 18.8149) (-1.551, 18.7306) (-1.5189, 18.6463) (-1.4872, 18.5619) (-1.4559, 18.4775) (-1.4249, 18.393) (-1.3943, 18.3084) (-1.3641, 18.2238) (-1.3344, 18.1391) (-1.305, 18.0543) (-1.276, 17.9694) (-1.2474, 17.8845) (-1.2215, 17.8065) (-1.2016, 17.7454) (-1.1873, 17.7013) (-1.1786, 17.6743) (-1.1754, 17.6642) knots -1 -1 -1 -1 -1 -1 -0.985714 -0.971429 -0.957143 -0.942857 -0.928571 -0.914286 -0.9 -0.885714 -0.871429 -0.857143 -0.842857 -0.828571 -0.814286 -0.8 -0.785714 -0.771429 -0.757143 -0.742857 -0.728571 -0.714286 -0.7 -0.685714 -0.671429 -0.657143 -0.642857 -0.628571 -0.614286 -0.6 -0.585714 -0.571429 -0.557143 -0.542857 -0.528571 -0.514286 -0.5 -0.485714 -0.471429 -0.457143 -0.442857 -0.428571 -0.414286 -0.405839 -0.405839 -0.405839 -0.405839 -0.405839 -0.405839
  arc A44 (0.1419, 17.7112) -> (-1.1754, 17.6642) centre (2.0032, -52.8695) ccw
  spline S45 degree 5 poles (0.1419, 17.7112) (0.1444, 17.7215) (0.1511, 17.7492) (0.1622, 17.7941) (0.1778, 17.8565) (0.198, 17.9362) (0.2205, 18.0229) (0.2433, 18.1096) (0.2666, 18.1962) (0.2903, 18.2829) (0.3143, 18.3694) (0.3388, 18.456) (0.3636, 18.5425) (0.3889, 18.6289) (0.4145, 18.7154) (0.4405, 18.8018) (0.4668, 18.8881) (0.4935, 18.9744) (0.5206, 19.0607) (0.548, 19.1469) (0.5758, 19.233) (0.604, 19.3192) (0.6325, 19.4053) (0.6613, 19.4913) (0.6905, 19.5773) (0.72, 19.6633) (0.7498, 19.7492) (0.78, 19.8351) (0.8105, 19.9209) (0.8414, 20.0067) (0.8726, 20.0924) (0.904, 20.1781) (0.9359, 20.2637) (0.968, 20.3493) (1.0004, 20.4348) (1.0332, 20.5203) (1.0663, 20.6058) (1.0996, 20.6912) (1.1333, 20.7765) (1.1673, 20.8618) (1.2016, 20.9471) (1.2362, 21.0323) (1.2711, 21.1174) (1.2992, 21.1855) (1.3205, 21.2366) (1.3347, 21.2706) (1.3418, 21.2876) knots 0.405839 0.405839 0.405839 0.405839 0.405839 0.405839 0.414286 0.428571 0.442857 0.457143 0.471429 0.485714 0.5 0.514286 0.528571 0.542857 0.557143 0.571429 0.585714 0.6 0.614286 0.628571 0.642857 0.657143 0.671429 0.685714 0.7 0.714286 0.728571 0.742857 0.757143 0.771429 0.785714 0.8 0.814286 0.828571 0.842857 0.857143 0.871429 0.885714 0.9 0.914286 0.928571 0.942857 0.957143 0.971429 0.985714 1 1 1 1 1 1
  arc A45 (2.6646, 21.2876) -> (1.3418, 21.2876) centre (2.0032, -52.8695) ccw
  spline S46 degree 5 poles (2.6646, 21.2876) (2.6717, 21.2706) (2.686, 21.2366) (2.7072, 21.1855) (2.7354, 21.1174) (2.7702, 21.0323) (2.8048, 20.9471) (2.8391, 20.8618) (2.8731, 20.7765) (2.9068, 20.6912) (2.9402, 20.6058) (2.9732, 20.5203) (3.006, 20.4348) (3.0384, 20.3493) (3.0706, 20.2637) (3.1024, 20.1781) (3.1339, 20.0924) (3.165, 20.0067) (3.1959, 19.9209) (3.2264, 19.8351) (3.2566, 19.7492) (3.2864, 19.6633) (3.316, 19.5773) (3.3451, 19.4913) (3.374, 19.4053) (3.4025, 19.3192) (3.4306, 19.233) (3.4584, 19.1469) (3.4858, 19.0607) (3.5129, 18.9744) (3.5396, 18.8881) (3.566, 18.8018) (3.592, 18.7154) (3.6176, 18.6289) (3.6428, 18.5425) (3.6676, 18.456) (3.6921, 18.3694) (3.7162, 18.2829) (3.7398, 18.1962) (3.7631, 18.1096) (3.786, 18.0229) (3.8084, 17.9362) (3.8287, 17.8565) (3.8442, 17.7941) (3.8553, 17.7492) (3.862, 17.7215) (3.8645, 17.7112) knots -1 -1 -1 -1 -1 -1 -0.985714 -0.971429 -0.957143 -0.942857 -0.928571 -0.914286 -0.9 -0.885714 -0.871429 -0.857143 -0.842857 -0.828571 -0.814286 -0.8 -0.785714 -0.771429 -0.757143 -0.742857 -0.728571 -0.714286 -0.7 -0.685714 -0.671429 -0.657143 -0.642857 -0.628571 -0.614286 -0.6 -0.585714 -0.571429 -0.557143 -0.542857 -0.528571 -0.514286 -0.5 -0.485714 -0.471429 -0.457143 -0.442857 -0.428571 -0.414286 -0.405839 -0.405839 -0.405839 -0.405839 -0.405839 -0.405839
  arc A46 (5.1818, 17.6642) -> (3.8645, 17.7112) centre (2.0032, -52.8695) ccw
  spline S47 degree 5 poles (5.1818, 17.6642) (5.185, 17.6743) (5.1937, 17.7013) (5.208, 17.7454) (5.228, 17.8065) (5.2538, 17.8845) (5.2824, 17.9694) (5.3114, 18.0543) (5.3408, 18.1391) (5.3706, 18.2238) (5.4008, 18.3084) (5.4313, 18.393) (5.4623, 18.4775) (5.4936, 18.5619) (5.5253, 18.6463) (5.5574, 18.7306) (5.5898, 18.8149) (5.6227, 18.899) (5.6558, 18.9832) (5.6893, 19.0672) (5.7232, 19.1512) (5.7574, 19.2351) (5.792, 19.3189) (5.8269, 19.4027) (5.8621, 19.4864) (5.8977, 19.57) (5.9336, 19.6536) (5.9698, 19.7371) (6.0064, 19.8205) (6.0433, 19.9039) (6.0805, 19.9871) (6.118, 20.0704) (6.1558, 20.1535) (6.194, 20.2366) (6.2325, 20.3196) (6.2712, 20.4025) (6.3103, 20.4854) (6.3497, 20.5682) (6.3894, 20.6509) (6.4294, 20.7336) (6.4697, 20.8162) (6.5102, 20.8987) (6.5511, 20.9812) (6.584, 21.0471) (6.6089, 21.0964) (6.6255, 21.1294) (6.6338, 21.1458) knots 0.405839 0.405839 0.405839 0.405839 0.405839 0.405839 0.414286 0.428571 0.442857 0.457143 0.471429 0.485714 0.5 0.514286 0.528571 0.542857 0.557143 0.571429 0.585714 0.6 0.614286 0.628571 0.642857 0.657143 0.671429 0.685714 0.7 0.714286 0.728571 0.742857 0.757143 0.771429 0.785714 0.8 0.814286 0.828571 0.842857 0.857143 0.871429 0.885714 0.9 0.914286 0.928571 0.942857 0.957143 0.971429 0.985714 1 1 1 1 1 1
  arc A47 (7.9532, 21.0514) -> (6.6338, 21.1458) centre (2.0032, -52.8695) ccw